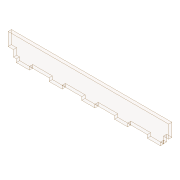
# Autodesk Inventor part: Divisória-24cm
Saved by Autodesk Inventor 2020 (Build 240168000, 168)
## iProperties
Created: 2021-09-22
Part Number: Divisória-24cm
Material: Generic
Document SubType Name: Modeling
Designer: pablo
Density: 1 g/cm^3
Appearance: Polycarbonate - Smoked
Author: pablo
Autodesk Inventor part; units mm, degrees
ref_plane "YZ Plane" through (0, 0, 0) normal (1, 0, 0) x (0, 1, 0)
ref_plane "XZ Plane" through (0, 0, 0) normal (0, 1, 0) x (-1, 0, 0)
ref_plane "XY Plane" through (0, 0, 0) normal (0, 0, 1) x (1, 0, 0)
sketch "Sketch1" plane through (0, 0, 0) normal (0, 0, 1) x (1, 0, 0)
  line L0 (-122.5, 15) -> (122.5, 15)
  line L1 (122.5, 15) -> (122.5, -15)
  line L2 (122.5, -15) -> (-122.5, -15)
  line L3 (-122.5, -15) -> (-122.5, 15)
  line L4 (-122.5, 15) -> (122.5, -15) construction
  line L5 (122.5, 15) -> (-122.5, -15) construction
  point P0 (0, 0)
  dimension "d0" = 30
  dimension "d1" = 245
  constraints: 12 end point, 2 midpoint, 2 parallel, 1 horizontal, 1 perpendicular
  measures "d0" distance of L0.end L1.end
  measures "d1" distance of L1.end L2.end
extrude "Extrusion1" add sketch "Sketch1" along normal blind 5
sketch "Sketch2" plane through (0, 0, 5) normal (0, 0, 1) x (1, 0, 0)
  line L0 (-110, -14.8732) -> (-90, -14.8732)
  line L1 (-90, -14.8732) -> (-90, -19.8732)
  line L2 (-90, -19.8732) -> (-110, -19.8732)
  line L3 (-110, -19.8732) -> (-110, -14.8732)
  line L4 (-122.5, 15) -> (-122.5, -15) projected
  line L5 (-60, -14.8732) -> (-40, -14.8732)
  line L6 (-40, -14.8732) -> (-40, -19.8732)
  line L7 (-40, -19.8732) -> (-60, -19.8732)
  line L8 (-60, -19.8732) -> (-60, -14.8732)
  line L9 (-10, -14.8732) -> (10, -14.8732)
  line L10 (10, -14.8732) -> (10, -19.8732)
  line L11 (10, -19.8732) -> (-10, -19.8732)
  line L12 (-10, -19.8732) -> (-10, -14.8732)
  line L13 (40, -14.8732) -> (60, -14.8732)
  line L14 (60, -14.8732) -> (60, -19.8732)
  line L15 (60, -19.8732) -> (40, -19.8732)
  line L16 (40, -19.8732) -> (40, -14.8732)
  line L17 (90, -14.8732) -> (110, -14.8732)
  line L18 (110, -14.8732) -> (110, -19.8732)
  line L19 (110, -19.8732) -> (90, -19.8732)
  line L20 (90, -19.8732) -> (90, -14.8732)
  point P0 (0, 0)
  dimension "d4" = 20
  dimension "d5" = 5
  dimension "d6" = 12.5
  dimension "d9" = 50
  constraints: 40 end point, 2 horizontal, 2 parallel, 1 collinear, 1 perpendicular, 31 other
  measures "d4" distance of L1.end L2.end
  measures "d5" distance of L0.end L1.end
  measures "d6" distance from line of L4 L0.start
  measures "d9" distance of L0.start L5.start
extrude "Extrusion2" add sketch "Sketch2" against normal blind 5
sketch "Sketch3" plane through (0, 0, 5) normal (0, 0, 1) x (1, 0, 0)
  line L0 (-122.5, 15) -> (-122.5, -15) projected
  line L1 (-122.5, -15) -> (-114.5, -15)
  line L2 (-114.5, -15) -> (-114.5, -5)
  line L3 (-114.5, -5) -> (-122.5, -5)
  line L4 (-122.5, -5) -> (-122.5, -15)
  line L5 (0, 0) -> (0, -7.9678)
  line L6 (122.5, -15) -> (114.5, -15)
  line L7 (114.5, -15) -> (114.5, -5)
  line L8 (114.5, -5) -> (122.5, -5)
  line L9 (122.5, -5) -> (122.5, -15)
  dimension "d18" = 8
  dimension "d19" = 10
  constraints: 18 end point, 4 symmetric about line, 2 parallel, 1 horizontal, 1 perpendicular, 1 vertical
  measures "d18" distance of L3.end L2.end
  measures "d19" distance of L2.end L1.end
extrude "Extrusion3" cut sketch "Sketch3" against normal blind 5
body "Solid1"
